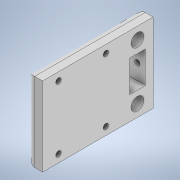
# Autodesk Inventor part: Joint_Tubes_1_3
Saved by Autodesk Inventor 2022.3 (Build 263350000, 350)
## iProperties
Created: 2023-05-15
Part Number: Joint_Tubes_1_3
Material: Generic
Document SubType Name: Modeling
Designer: Manuel Hueso Béjar
Density: 1 g/cm^3
Appearance: Default
Author: Manuel Hueso Béjar
Autodesk Inventor part; units mm, degrees
ref_plane "YZ Plane" through (0, 0, 0) normal (1, 0, 0) x (0, 1, 0)
ref_plane "XZ Plane" through (0, 0, 0) normal (0, 1, 0) x (-1, 0, 0)
ref_plane "XY Plane" through (0, 0, 0) normal (0, 0, 1) x (1, 0, 0)
sketch "Sketch1" plane through (0, 0, 0) normal (0, 1, 0) x (-1, 0, 0)
  line L0 (-5, 35) -> (5, 35)
  line L1 (5, 35) -> (5, -35)
  line L2 (5, -35) -> (-5, -35)
  line L3 (-5, -35) -> (-5, 35)
  line L4 (-5, 35) -> (5, -35) construction
  line L5 (5, 35) -> (-5, -35) construction
  point P0 (0, 0)
  dimension "d0" = 10
  dimension "d1" = 70
  constraints: 12 end point, 2 midpoint, 2 parallel, 1 horizontal, 1 perpendicular
  measures "d0" distance of L1.end L2.end
  measures "d1" distance of L0.end L1.end
extrude "Extrusion1" add sketch "Sketch1" along normal blind 50
sketch "Sketch2" plane through (-5, 0, -35) normal (-1, 0, 0) x (0, 0, 1)
  line L0 (0, 0) -> (70, 0) projected
  line L1 (0, 50) -> (20, 50)
  line L2 (20, 50) -> (20, 0)
  line L3 (20, 0) -> (0, 0)
  line L4 (0, 0) -> (0, 50)
  line L5 (0, 50) -> (70, 50) projected
  line L6 (10, 50) -> (10, 42.5)
  line L7 (10, 0) -> (10, 7.5)
  line L8 (10, 0) -> (17.5, 0) construction
  circle A0 centre (10, 42.5) radius 4.1
  circle A1 centre (10, 42.5) radius 6
  circle A2 centre (10, 7.5) radius 4.1
  circle A3 centre (10, 7.5) radius 6
  line L9 (70, 0) -> (0, 0) projected
  line L10 (5, 15) -> (15, 15)
  line L11 (15, 15) -> (15, 35)
  line L12 (15, 35) -> (5, 35)
  line L13 (5, 35) -> (5, 15)
  line L14 (5, 15) -> (15, 35) construction
  line L15 (15, 15) -> (5, 35) construction
  point P0 (35, 0)
  point P1 (10, 25)
  dimension "d4" = 20
  dimension "d5" = 7.5
  dimension "d6" = 7.5
  dimension "d7" = 90
  dimension "d8" = 8.2
  dimension "d9" = 12
  dimension "d10" = 8.2
  dimension "d11" = 12
  dimension "d12" = 10
  dimension "d13" = 20
  constraints: 26 end point, 4 centre point, 4 coincident, 4 parallel, 4 perpendicular, 3 horizontal, 3 midpoint, 2 point on line, 1 vertical
  measures "d4" distance of L2.end L3.end
  measures "d5" distance of L6.start L6.end
  measures "d6" distance of L7.start L7.end
  measures "d7" angle of L8 L7
  measures "d8" diameter of A0
  measures "d9" diameter of A1
  measures "d10" diameter of A2
  measures "d11" diameter of A3
  measures "d12" distance of L12.end L11.end
  measures "d13" distance of L11.end L10.end
extrude "Extrusion2" cut sketch "Sketch2" against normal through all contours A0 | A2 | L13 L12 L11 L10
extrude "Extrusion3" cut sketch "Sketch2" against normal blind 2 contours A1 | A3
sketch "Sketch3" plane through (-5, 0, -35) normal (-1, 0, 0) x (0, 0, 1)
  line L0 (70, 0) -> (70, 50) projected
  line L1 (70, 50) -> (60, 50)
  line L2 (60, 50) -> (60, 45)
  line L3 (60, 45) -> (70, 45)
  line L4 (70, 45) -> (70, 50)
  line L5 (60, 45) -> (30, 45)
  line L6 (30, 45) -> (30, 5)
  line L7 (30, 5) -> (60, 5)
  line L8 (60, 5) -> (60, 45)
  point P0 (35, 0)
  dimension "d18" = 10
  dimension "d19" = 5
  dimension "d20" = 30
  dimension "d21" = 40
  constraints: 16 end point, 4 parallel, 2 horizontal, 2 perpendicular
  measures "d18" distance of L3.end L2.end
  measures "d19" distance of L2.end L1.end
  measures "d20" distance of L7.end L6.end
  measures "d21" distance of L6.end L5.end
hole "Hole1" at (-5, 45, 25) at (-5, 45, -5) at (-5, 5, -5) at (-5, 5, 25) direction (1, 0, 0) diameter 3.4 end through all countersink diameter 5.9 countersink angle 90
sketch "Sketch4" plane through (5, 0, -35) normal (0, 0, -1) x (-1, 0, 0)
  line L0 (0, 15) -> (0, 35) projected
  line L1 (0, 0) -> (0, 50) projected
  line L2 (0, 25) -> (10, 25)
  line L3 (10, 0) -> (10, 50) projected
  line L4 (5, 25) -> (5, 20)
  line L5 (5, 25) -> (10, 25) construction
  point P0 (5, 0)
  dimension "d30" = 5
  dimension "d31" = 90
  constraints: 6 end point, 3 midpoint, 1 horizontal, 1 perpendicular, 1 vertical
  measures "d30" distance of L4.start L4.end
  measures "d31" angle of L4 L5
fillet "Fillet1" radius 5 4 edges at (-5, 50, 0) (-5, 25, -35) (-5, 0, 0) (-5, 25, 35)
hole "Hole2" at (0, 25, -35) direction (0, 0, 1) diameter 3.4 depth 5 countersink diameter 5.9 countersink angle 90
sketch "Sketch5" plane through (-5, 15, -20) normal (0, 0, -1) x (-1, 0, 0)
  line L0 (-10, 0) -> (-10, 20) projected
  line L1 (0, 20) -> (-10, 20) projected
  line L2 (-10, 0) -> (0, 20)
  line L3 (-5, 10) -> (-10, 10)
  point P0 (-5, -15)
  constraints: 4 end point, 2 midpoint
hole "Hole3" at (0, 25, -20) direction (0, 0, 1) diameter 3.4 depth 12 counterbore diameter 4.1 counterbore depth 5.1
sketch "Sketch6" plane through (-5, 15, -20) normal (-1, 0, 0) x (0, 0, 1)
  line L0 (50, -10) -> (0, -10) construction
  line L1 (0, -10) -> (0, 30) construction
  line L2 (0, 30) -> (50, 30) construction
  line L3 (50, 30) -> (50, -10) construction
  line L4 (50, 30) -> (50, -10) projected
  line L5 (42.05, -10) -> (17.95, -10) projected
  line L6 (43.1605, 15) -> (39.7893, 5)
  line L7 (39.7893, 5) -> (38.1523, 5)
  line L8 (38.1523, 5) -> (34.7812, 15)
  line L9 (34.7812, 15) -> (36.1831, 15)
  line L10 (36.1831, 15) -> (37.0908, 12.2042)
  line L11 (37.0908, 12.2042) -> (40.9076, 12.2042)
  line L12 (40.9076, 12.2042) -> (41.8152, 15)
  line L13 (41.8152, 15) -> (43.1605, 15)
  line L14 (37.4554, 11.0697) -> (39.0032, 6.3614)
  line L15 (39.0032, 6.3614) -> (40.5429, 11.0697)
  line L16 (40.5429, 11.0697) -> (37.4554, 11.0697)
  line L17 (28.0389, 15) -> (33.8331, 15)
  line L18 (33.8331, 15) -> (33.8331, 5)
  line L19 (33.8331, 5) -> (32.5041, 5)
  line L20 (32.5041, 5) -> (32.5041, 13.8169)
  line L21 (32.5041, 13.8169) -> (28.0389, 13.8169)
  line L22 (28.0389, 13.8169) -> (28.0389, 15)
  line L23 (23.5089, 15) -> (27.3825, 15)
  line L24 (27.3825, 15) -> (27.3825, 13.9789)
  line L25 (27.3825, 13.9789) -> (26.1102, 13.9789)
  line L26 (26.1102, 13.9789) -> (26.1102, 6.0211)
  line L27 (26.1102, 6.0211) -> (27.3825, 6.0211)
  line L28 (27.3825, 6.0211) -> (27.3825, 5)
  line L29 (27.3825, 5) -> (23.5089, 5)
  line L30 (23.5089, 5) -> (23.5089, 6.0211)
  line L31 (23.5089, 6.0211) -> (24.7812, 6.0211)
  line L32 (24.7812, 6.0211) -> (24.7812, 13.9789)
  line L33 (24.7812, 13.9789) -> (23.5089, 13.9789)
  line L34 (23.5089, 13.9789) -> (23.5089, 15)
  spline S0 degree 2 poles (17.9579, 15.1783) (18.9303, 15.1783) (20.5754, 14.5219) (21.175, 13.8655) knots 0 0 0 1 2 2 2
  spline S1 degree 2 poles (21.175, 13.8655) (21.7747, 13.2172) (22.4311, 11.2723) (22.4311, 10.0081) knots 0 0 0 1 2 2 2
  spline S2 degree 2 poles (22.4311, 10.0081) (22.4311, 8.752) (21.7909, 6.8882) (21.1831, 6.1994) knots 0 0 0 1 2 2 2
  spline S3 degree 2 poles (21.1831, 6.1994) (20.5835, 5.5267) (18.9465, 4.8217) (17.9335, 4.8217) knots 0 0 0 1 2 2 2
  spline S4 degree 2 poles (17.9335, 4.8217) (17.4311, 4.8217) (16.5478, 4.9676) (16.175, 5.081) knots 0 0 0 1 2 2 2
  spline S5 degree 2 poles (16.175, 5.081) (15.8509, 5.1864) (15.1783, 5.4862) (14.846, 5.6645) knots 0 0 0 1 2 2 2
  line L35 (14.846, 5.6645) -> (14.846, 7.269)
  line L36 (14.846, 7.269) -> (14.9514, 7.269)
  spline S6 degree 2 poles (14.9514, 7.269) (15.1297, 7.107) (15.6807, 6.6532) (16.0778, 6.4344) knots 0 0 0 1 2 2 2
  spline S7 degree 2 poles (16.0778, 6.4344) (16.4587, 6.2237) (17.3582, 5.9562) (17.9417, 5.9562) knots 0 0 0 1 2 2 2
  spline S8 degree 2 poles (17.9417, 5.9562) (18.5818, 5.9562) (19.7245, 6.483) (20.154, 6.9854) knots 0 0 0 1 2 2 2
  spline S9 degree 2 poles (20.154, 6.9854) (20.5754, 7.4959) (21.0454, 9.0438) (21.0454, 10.0081) knots 0 0 0 1 2 2 2
  spline S10 degree 2 poles (21.0454, 10.0081) (21.0454, 11.0373) (20.5511, 12.5203) (20.1216, 13.0308) knots 0 0 0 1 2 2 2
  spline S11 degree 2 poles (20.1216, 13.0308) (19.7002, 13.5251) (18.5737, 14.0276) (17.9417, 14.0276) knots 0 0 0 1 2 2 2
  spline S12 degree 2 poles (17.9417, 14.0276) (17.3663, 14.0276) (16.3857, 13.7439) (16.0049, 13.5332) knots 0 0 0 1 2 2 2
  spline S13 degree 2 poles (16.0049, 13.5332) (15.6402, 13.3225) (15.0972, 12.8849) (14.9433, 12.731) knots 0 0 0 1 2 2 2
  line L37 (14.9433, 12.731) -> (14.846, 12.731)
  line L38 (14.846, 12.731) -> (14.846, 14.3193)
  spline S14 degree 2 poles (14.846, 14.3193) (15.1783, 14.4733) (15.7617, 14.7569) (16.175, 14.8865) knots 0 0 0 1 2 2 2
  spline S15 degree 2 poles (16.175, 14.8865) (16.6126, 15.0324) (17.3582, 15.1783) (17.9579, 15.1783) knots 0 0 0 1 2 2 2
  line L39 (13.6062, 15) -> (13.6062, 5)
  line L40 (13.6062, 5) -> (7.3501, 5)
  line L41 (7.3501, 5) -> (7.3501, 6.1831)
  line L42 (7.3501, 6.1831) -> (12.2771, 6.1831)
  line L43 (12.2771, 6.1831) -> (12.2771, 8.9222)
  line L44 (12.2771, 8.9222) -> (7.6823, 8.9222)
  line L45 (7.6823, 8.9222) -> (7.6823, 10.1053)
  line L46 (7.6823, 10.1053) -> (12.2771, 10.1053)
  line L47 (12.2771, 10.1053) -> (12.2771, 13.8169)
  line L48 (12.2771, 13.8169) -> (7.3501, 13.8169)
  line L49 (7.3501, 13.8169) -> (7.3501, 15)
  line L50 (7.3501, 15) -> (13.6062, 15)
  point P0 (20, -15)
  dimension "d46" = 40
  dimension "d47" = 0
  dimension "d48" = 50
  dimension "d49" = 0
  constraints: 2 other
  measures "d46" distance of L2.end L0.start
  measures "d47" distance between parallel lines of L4 L3
  measures "d48" distance of L0.start L0.end
  measures "d49" distance between parallel lines of L5 L0
emboss "Emboss1" sketch "Sketch6" operation cut depth 1 direction (1, 0, 0)
body "Solid1"
